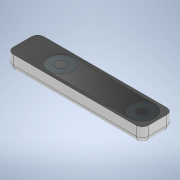
# Autodesk Inventor part: IntelRealSenseT265
Saved by Autodesk Inventor 2020 (Build 240168000, 168)
## iProperties
Created: 2020-02-28
Part Number: IntelRealSenseT265
Material: Generic
Document SubType Name: Modeling
Designer: Cooper
Density: 1 g/cm^3
Appearance: Default
Author: Cooper
Autodesk Inventor part; units mm, degrees
ref_plane "YZ Plane" through (0, 0, 0) normal (1, 0, 0) x (0, 1, 0)
ref_plane "XZ Plane" through (0, 0, 0) normal (0, 1, 0) x (-1, 0, 0)
ref_plane "XY Plane" through (0, 0, 0) normal (0, 0, 1) x (1, 0, 0)
sketch "Sketch1" plane through (0, 0, 0) normal (0, 1, 0) x (-1, 0, 0)
  line L0 (0, 0) -> (0, -12.25)
  line L1 (0, -12.25) -> (54, -12.25)
  line L2 (54, -12.25) -> (54, 12.25)
  line L3 (54, 12.25) -> (-54, 12.25)
  line L4 (-54, 12.25) -> (-54, -12.25)
  line L5 (-54, -12.25) -> (0, -12.25)
  dimension "d0" = 12.25
  dimension "d1" = 54
  dimension "d2" = 24.5
  dimension "d3" = 108
  dimension "d4" = 24.5
  constraints: 12 end point, 3 perpendicular, 1 collinear, 1 point on line, 1 vertical
  measures "d0" distance of L0.start L0.end
  measures "d1" distance of L0.end L1.end
  measures "d2" distance of L1.end L2.end
  measures "d3" distance of L2.end L3.end
  measures "d4" distance of L3.end L4.end
extrude "Extrusion1" add sketch "Sketch1" along normal blind 12.5
fillet "Fillet1" radius 5 4 edges at (-54, 6.25, 12.25) (-54, 6.25, -12.25) (54, 6.25, 12.25) (54, 6.25, -12.25)
sketch "Sketch2" plane through (0, 12.5, 0) normal (0, 1, 0) x (1, 0, 0)
  line L0 (54, -7.25) -> (54, 7.25) projected
  line L1 (54, 0) -> (41.75, 0)
  circle A0 centre (41.75, 0) radius 10
  line L2 (41.75, 0) -> (-23.25, 0)
  circle A1 centre (-23.25, 0) radius 10
  line L3 (-23.25, 10) -> (41.75, 10)
  line L4 (-23.25, -10) -> (41.75, -10)
  point P0 (0, 0)
  dimension "d8" = 12.25
  dimension "d9" = 20
  dimension "d10" = 65
  dimension "d11" = 20
  constraints: 8 end point, 4 point on circle, 2 centre point, 2 coincident, 2 horizontal, 2 tangent, 1 midpoint
  measures "d8" distance of L1.start L1.end
  measures "d9" diameter of A0
  measures "d10" distance of L2.start L2.end
  measures "d11" diameter of A1
extrude "Extrusion2" cut sketch "Sketch2" against normal blind 0.1
sketch "Sketch3" plane through (0, 12.4, 0) normal (0, 1, 0) x (1, 0, 0)
  line L0 (-23.25, 10) -> (41.75, 10) projected
  arc A0 (-23.25, 10) -> (-23.25, -10) centre (-23.25, 0) ccw projected
  line L1 (41.75, -10) -> (-23.25, -10) projected
  arc A1 (41.75, -10) -> (41.75, 10) centre (41.75, 0) ccw projected
  circle A2 centre (-23.25, 0) radius 9.5
  circle A3 centre (41.75, 0) radius 9.5
  point P0 (0, 0)
  dimension "d14" = 19
  dimension "d15" = 19
  constraints: 2 centre point, 2 coincident
  measures "d14" diameter of A2
  measures "d15" diameter of A3
extrude "Extrusion3" cut sketch "Sketch3" against normal blind 0.1 contours A2 | A3
sketch "Sketch4" plane through (-23.25, 12.3, 0) normal (0, 1, 0) x (1, 0, 0)
  circle A0 centre (0, 0) radius 9.5 projected
  circle A1 centre (65, 0) radius 9.5 projected
  circle A2 centre (0, 0) radius 4
  circle A3 centre (65, 0) radius 4
  point P0 (23.25, 0)
  dimension "d18" = 8
  dimension "d19" = 8
  constraints: 2 centre point, 2 coincident
  measures "d18" diameter of A2
  measures "d19" diameter of A3
extrude "Extrusion4" add sketch "Sketch4" along normal blind 0.1 contours A2 | A3
fillet "Fillet2" radius 5 8 edges at (-52.5355, 0, -10.7855) (-54, 0, 0) (-52.5355, 0, 10.7855) (0, 0, 12.25) (52.5355, 0, 10.7855) (54, 0, 0) (52.5355, 0, -10.7855) (0, 0, -12.25)
sketch "Sketch5" plane through (0, 0, 0) normal (0, -1, 0) x (1, 0, 0)
  line L0 (0, 0) -> (-25, 0)
  line L1 (0, 0) -> (25, 0)
  circle A0 centre (25, 0) radius 1.5
  circle A1 centre (-25, 0) radius 1.5
  dimension "d23" = 25
  dimension "d24" = 25
  dimension "d25" = 3
  dimension "d26" = 3
  constraints: 4 end point, 2 centre point, 2 coincident, 2 horizontal
  measures "d23" distance of L0.start L0.end
  measures "d24" distance of L0.start L1.end
  measures "d25" diameter of A0
  measures "d26" diameter of A1
extrude "Extrusion5" cut sketch "Sketch5" against normal blind 2
body "Solid1"
